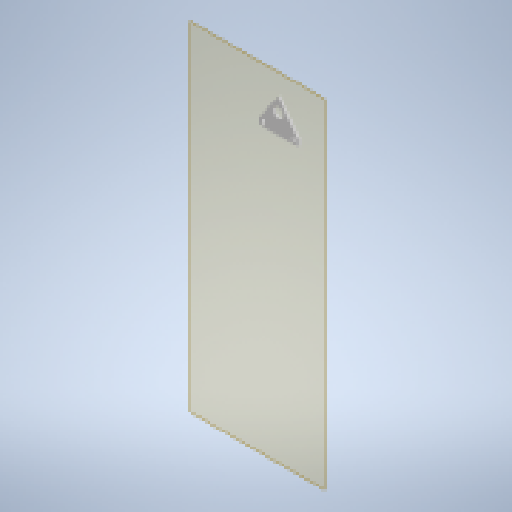
# Autodesk Inventor part: крепеж подшипника
Saved by Autodesk Inventor 2024.2 (Build 282272000, 272)
## iProperties
Created: 2026-03-04
Part Number: крепеж подшипника
Material: Типовые
Document SubType Name: Modeling
Designer: Service
Density: 1 g/cm^3
Appearance: По умолчанию
Author: Service
Autodesk Inventor part; units mm, degrees
ref_plane "YZ Plane" through (0, 0, 0) normal (1, 0, 0) x (0, 1, 0)
ref_plane "XZ Plane" through (0, 0, 0) normal (0, 1, 0) x (-1, 0, 0)
ref_plane "XY Plane" through (0, 0, 0) normal (0, 0, 1) x (1, 0, 0)
ref_plane "РабПлоскость1" through (0, 0, 0) normal (0, 0, 1) x (1, 0, 0)
sketch "Эскиз1" plane through (0, 0, 0) normal (0, 0, 1) x (1, 0, 0)
  line L0 (1.0452, 115.4021) -> (1.0452, 120.0556)
  line L1 (1.0452, 120.0556) -> (17.9158, 143.9758)
  line L2 (17.9158, 143.9758) -> (34.7864, 120.0556)
  line L3 (34.7864, 120.0556) -> (34.7864, 115.4021)
  line L4 (34.7864, 115.4021) -> (1.0452, 115.4021)
  circle A0 centre (5, 119) radius 1.5 projected
  circle A1 centre (31, 119) radius 1.5 projected
  circle A2 centre (17.9158, 132.0157) radius 4.1064
  point P0 (0, 0)
  constraints: 10 end point, 2 equal length, 1 centre point, 1 parallel, 1 perpendicular, 1 vertical
extrude "Выдавливание1" add sketch "Эскиз1" along normal blind 2
